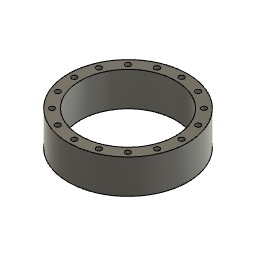
Untitled v2 (Autodesk Fusion 360 design; units mm, degrees)
Autodesk Fusion 360 part; units mm, degrees
note: some values were not read from the file. Set by a fixed rule: which sketch regions a step uses.
sketch "Sketch1" plane through (0, 0, 0) normal (0, 1, 0) x (1, 0, 0)
  circle A0 centre (0, 0) radius 17.5
  circle A1 centre (0, 0) radius 14
  dimension "d1" = 35
  dimension "d2" = 28
  constraint coincident A0.centre A1.centre
  measures "d1" diameter of A0
  measures "d2" diameter of A1
extrude "Extrude1" add sketch "Sketch1" along normal blind 10
sketch "Sketch2" plane through (0, 10, 0) normal (0, 1, 0) x (-1, 0, 0)
  circle A0 centre (0, 0) radius 14
  circle A1 centre (0, 0) radius 17.5
  line L0 (-14, -0.0032) -> (-17.5, -0.0032)
  circle A2 centre (-15.75, -0.0032) radius 0.75
  dimension "d5" = 3.5
  dimension "d6" = 1.5
  constraint coincident A0 L0.start
  constraint coincident A1 L0.end
  constraint horizontal L0
  constraint midpoint L0 A2.centre
  measures "d5" distance of L0.start L0.end
  measures "d6" diameter of A2
extrude "Extrude2" cut sketch "Sketch2" against normal blind 10 contours L0 A2 | L0 A2
pattern_circular "C-Pattern1" count 16 over 360 about axis through (0, 1.75, 0) along (0, 1, 0) of "Extrude2"
